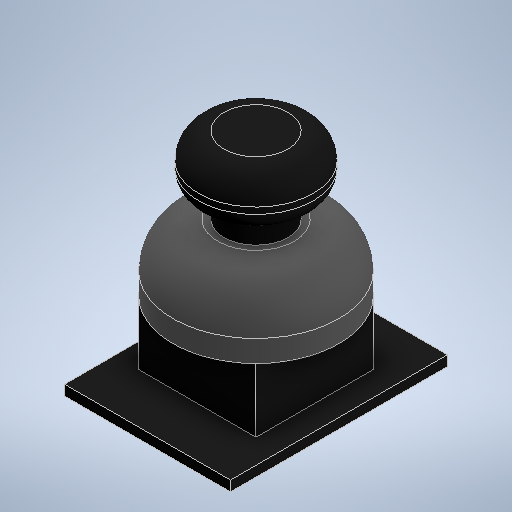
# Autodesk Inventor part: stick
Saved by Autodesk Inventor 2026.1 (Build 301233020, 233B)
## iProperties
Created: 2026-01-20
Part Number: stick
Material: 一般
Document SubType Name: Modeling
Designer: hibik
Density: 1 g/cm^3
Appearance: 既定
Author: hibik
Autodesk Inventor part; units mm, degrees
ref_plane "YZ Plane" through (0, 0, 0) normal (1, 0, 0) x (0, 1, 0)
ref_plane "XZ Plane" through (0, 0, 0) normal (0, 1, 0) x (-1, 0, 0)
ref_plane "XY Plane" through (0, 0, 0) normal (0, 0, 1) x (1, 0, 0)
sketch "スケッチ1" plane through (0, 0, 0) normal (0, 1, 0) x (-1, 0, 0)
  line L0 (13, 17) -> (-13, 17)
  line L1 (-13, 17) -> (-13, -17)
  line L2 (-13, -17) -> (13, -17)
  line L3 (13, -17) -> (13, 17)
  point P0 (0, 0)
  point P1 (0, 17)
  point P2 (13, 0)
  dimension "d0" = 34
  dimension "d1" = 26
  constraints: 8 end point, 2 midpoint, 2 parallel, 1 horizontal, 1 horizontal alignment, 1 perpendicular, 1 vertical alignment
  measures "d0" distance of L2.end L0.start
  measures "d1" distance of L0.start L0.end
extrude "押し出し1" add sketch "スケッチ1" along normal blind 1.6
sketch "スケッチ2" plane through (0, 0, 0) normal (0, -1, 0) x (1, 0, 0)
  circle A0 centre (0, 0) radius 13
  line L0 (13, 17) -> (13, -17) projected
  constraints: 1 centre point, 1 coincident, 1 tangent
extrude "押し出し2" add sketch "スケッチ2" against normal blind 22
sketch "スケッチ3" plane through (0, 22, 0) normal (0, 1, 0) x (1, 0, 0)
  circle A0 centre (0, 0) radius 5
  dimension "d6" = 10
  constraints: 1 centre point, 1 coincident
  measures "d6" diameter of A0
extrude "押し出し3" add sketch "スケッチ3" along normal blind 12
sketch "スケッチ4" plane through (0, 34, 0) normal (0, 1, 0) x (1, 0, 0)
  circle A0 centre (0, 0) radius 9
  dimension "d9" = 18
  constraints: 1 centre point, 1 coincident
  measures "d9" diameter of A0
extrude "押し出し4" add sketch "スケッチ4" against normal blind 8
sketch "スケッチ5" plane through (0, 1.6, 0) normal (0, 1, 0) x (1, 0, 0)
  circle A0 centre (0, 0) radius 13 projected
  line L0 (-9.1924, -9.1924) -> (9.1924, -9.1924)
  line L1 (9.1924, -9.1924) -> (9.1924, 9.1924)
  line L2 (9.1924, 9.1924) -> (-9.1924, 9.1924)
  line L3 (-9.1924, 9.1924) -> (-9.1924, -9.1924)
  arc A1 (13, 0) -> (-13, 0) centre (0, 0) ccw projected
  arc A2 (-13, 0) -> (13, 0) centre (0, 0) ccw projected
  constraints: 8 end point, 3 point on circle, 2 parallel, 2 perpendicular, 1 horizontal
extrude "押し出し5" cut sketch "スケッチ5" along normal blind 10 contours A0 L1 | L2 A0 | A0 L0 | L3 A0
fillet "フィレット1" radius 7 1 edges at (-13, 22, 0)
fillet "フィレット2" radius 4 1 edges at (-9, 34, 0)
fillet "フィレット3" radius 3 1 edges at (-9, 26, 0)
